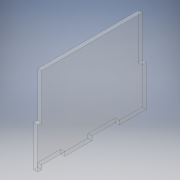
# Autodesk Inventor part: side
Saved by Autodesk Inventor 2017.2 (Build 212233000, 233)
## iProperties
Created: 2017-06-02
Part Number: side
Material: Generic
Document SubType Name: Modeling
Designer: SandeepSH
Density: 1 g/cm^3
Appearance: Polycarbonate - Clear
Author: SandeepSH
Autodesk Inventor part; units mm, degrees
ref_plane "YZ Plane" through (0, 0, 0) normal (1, 0, 0) x (0, 1, 0)
ref_plane "XZ Plane" through (0, 0, 0) normal (0, 1, 0) x (-1, 0, 0)
ref_plane "XY Plane" through (0, 0, 0) normal (0, 0, 1) x (1, 0, 0)
sketch "Sketch1" plane through (0, 0, 0) normal (1, 0, 0) x (0, 1, 0)
  line L0 (-31.5, 40) -> (31.5, 40)
  line L1 (31.5, 40) -> (31.5, -40)
  line L2 (31.5, -40) -> (-31.5, -40)
  line L3 (-31.5, -40) -> (-31.5, 40)
  line L4 (-31.5, 40) -> (31.5, -40) construction
  line L5 (31.5, 40) -> (-31.5, -40) construction
  point P0 (0, 0)
  dimension "d0" = 63
  dimension "d1" = 80
  constraints: 12 end point, 2 midpoint, 2 parallel, 1 horizontal, 1 perpendicular
  measures "d0" distance of L1.end L2.end
  measures "d1" distance of L0.end L1.end
extrude "Extrusion1" add sketch "Sketch1" along normal blind 3
sketch "Sketch2" plane through (3, 0, 0) normal (1, 0, 0) x (0, 0, -1)
  line L0 (40, -31.5) -> (40, 31.5) projected
  line L1 (40, 31.5) -> (37, 31.5)
  line L2 (37, 31.5) -> (37, -1.5)
  line L3 (37, -1.5) -> (40, -1.5)
  line L4 (40, -1.5) -> (40, 31.5)
  line L5 (-40, -31.5) -> (40, -31.5) projected
  line L6 (0, -31.5) -> (20, -31.5)
  line L7 (20, -31.5) -> (20, -28.5)
  line L8 (20, -28.5) -> (0, -28.5)
  line L9 (0, -28.5) -> (0, -31.5)
  line L10 (-37, -31.5) -> (-20, -31.5)
  line L11 (-20, -31.5) -> (-20, -28.5)
  line L12 (-20, -28.5) -> (-37, -28.5)
  line L13 (-37, -28.5) -> (-37, -31.5)
  point P0 (0, 0)
  dimension "d4" = 3
  dimension "d5" = 30
  dimension "d6" = 20
  dimension "d7" = 3
  dimension "d8" = 20
  dimension "d9" = 17
  dimension "d10" = 3
  dimension "d11" = 20
  constraints: 24 end point, 6 parallel, 3 horizontal, 3 perpendicular, 1 midpoint, 1 point on line
  measures "d4" distance of L3.end L2.end
  measures "d5" distance between parallel lines of L5 L3
  measures "d6" distance of L8.end L7.end
  measures "d7" distance of L7.end L6.end
  measures "d8" distance between parallel lines of L0 L7
  measures "d9" distance of L12.end L11.end
  measures "d10" distance of L11.end L10.end
  measures "d11" distance between parallel lines of L9 L11
extrude "Extrusion2" cut sketch "Sketch2" against normal through all
sketch "Sketch3" plane through (3, 0, 0) normal (1, 0, 0) x (0, 0, -1)
  line L0 (-40, 31.5) -> (-40, -31.5) projected
  line L1 (-40, 31.5) -> (-37, 31.5)
  line L2 (-37, 31.5) -> (-37, -1.5)
  line L3 (-37, -1.5) -> (-40, -1.5)
  line L4 (-40, -1.5) -> (-40, 31.5)
  point P0 (0, 0)
  dimension "d14" = 3
  dimension "d15" = 33
  constraints: 8 end point, 2 parallel, 1 horizontal, 1 perpendicular
  measures "d14" distance of L2.end L3.end
  measures "d15" distance of L1.end L2.end
extrude "Extrusion3" cut sketch "Sketch3" against normal through all
body "Solid1"
